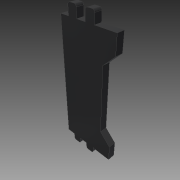
# Autodesk Inventor part: spool_stand_brace_middle_a
Saved by Autodesk Inventor 2014 (Build 180170000, 170)
## iProperties
Created: 2014-04-08
Part Number: spool_stand_brace_middle_a
Material: Plywood, Finish
Document SubType Name: Modeling
Designer: buben
Density: 0.552 g/cm^3
Appearance: Plywood - New
Author: buben
Autodesk Inventor part; units mm, degrees
ref_plane "YZ Plane" through (0, 0, 0) normal (1, 0, 0) x (0, 1, 0)
ref_plane "XZ Plane" through (0, 0, 0) normal (0, 1, 0) x (-1, 0, 0)
ref_plane "XY Plane" through (0, 0, 0) normal (0, 0, 1) x (1, 0, 0)
sketch "Sketch1" plane through (0, 0, 0) normal (0, 1, 0) x (-1, 0, 0)
  line L0 (0, 0) -> (-40, 0)
  line L1 (-40, 0) -> (-40, -110)
  line L2 (-40, -110) -> (0, -110)
  line L3 (0, -110) -> (0, 0)
  dimension "d0" = 110
  dimension "d1" = 40
  constraints: 8 end point, 2 parallel, 1 horizontal, 1 perpendicular
  measures "d0" distance of L2.end L0.start
  measures "d1" distance of L0.start L0.end
extrude "Extrusion1" add sketch "Sketch1" along normal blind 6.5
sketch "Sketch2" plane through (0, 6.5, 0) normal (0, 1, 0) x (1, 0, 0)
  line L0 (40, 0) -> (40, 110) projected
  line L1 (40, 110) -> (0, 110) projected
  line L2 (0, 110) -> (0, 0) projected
  line L3 (8, 110) -> (16, 110)
  line L4 (16, 110) -> (16, 114.5)
  line L5 (14, 116.5) -> (10, 116.5)
  line L6 (8, 114.5) -> (8, 110)
  line L7 (24, 110) -> (32, 110)
  line L8 (32, 110) -> (32, 114.5)
  line L9 (30, 116.5) -> (26, 116.5)
  line L10 (24, 114.5) -> (24, 110)
  arc A0 (10, 116.5) -> (8, 114.5) centre (10, 114.5) ccw
  arc A1 (16, 114.5) -> (14, 116.5) centre (14, 114.5) ccw
  arc A2 (26, 116.5) -> (24, 114.5) centre (26, 114.5) ccw
  arc A3 (32, 114.5) -> (30, 116.5) centre (30, 114.5) ccw
  line L11 (8, 112.25) -> (0, 112.25) construction
  line L12 (16, 112.25) -> (24, 112.25) construction
  line L13 (32, 112.25) -> (40, 112.25) construction
  line L14 (0, 55) -> (40, 55) construction
  line L15 (0, 0) -> (40, 0) projected
  line L16 (40, 0) -> (40, 110) projected
  line L17 (40, 110) -> (0, 110) projected
  line L18 (0, 110) -> (0, 0) projected
  line L19 (8, 0) -> (16, 0)
  line L20 (16, 0) -> (16, -7.5)
  line L21 (14, -9.5) -> (10, -9.5)
  line L22 (8, -7.5) -> (8, 0)
  line L23 (24, 0) -> (32, 0)
  line L24 (32, 0) -> (32, -7.5)
  line L25 (30, -9.5) -> (26, -9.5)
  line L26 (24, -7.5) -> (24, 0)
  arc A4 (8, -7.5) -> (10, -9.5) centre (10, -7.5) ccw
  arc A5 (14, -9.5) -> (16, -7.5) centre (14, -7.5) ccw
  arc A6 (24, -7.5) -> (26, -9.5) centre (26, -7.5) ccw
  arc A7 (30, -9.5) -> (32, -7.5) centre (30, -7.5) ccw
  dimension "d4" = 2
  dimension "d5" = 8
  dimension "d6" = 8
  dimension "d7" = 6.5
  dimension "d10" = 2
  dimension "d11" = 9.5
  constraints: 40 end point, 16 point on circle, 16 tangent, 9 collinear, 8 centre point, 8 parallel, 6 equal radius, 6 midpoint, 5 perpendicular, 4 horizontal, 4 point on line, 2 vertical alignment
  measures "d4" radius of A0
  measures "d5" distance between parallel lines of L4 L6
  measures "d6" distance between parallel lines of L8 L10
  measures "d7" distance between parallel lines of L3 L5
  measures "d10" radius of A4
  measures "d11" distance between parallel lines of L15 L21
extrude "Extrusion3" add sketch "Sketch2" against normal blind 6.5 contours L24 A7 L25 A6 L26 L15 | L1 L10 A2 L9 A3 L8 | L20 A5 L21 A4 L22 L15 | L1 L6 A0 L5 A1 L4
sketch "Sketch3" plane through (0, 0, 0) normal (0, -1, 0) x (1, 0, 0)
  line L0 (0, -110) -> (0, 0) projected
  line L1 (40, 0) -> (40, -110) projected
  line L2 (8, 7.5) -> (8, 0) projected
  line L3 (40, 0) -> (50, 0)
  line L4 (50, 0) -> (50, -15)
  line L5 (50, -15) -> (40, -25)
  line L6 (40, -85) -> (50, -95)
  line L7 (50, -95) -> (50, -110)
  line L8 (50, -110) -> (40, -110)
  line L9 (40, -85) -> (40, -110)
  line L10 (40, 0) -> (40, -25)
  dimension "d14" = 10
  dimension "d15" = 15
  dimension "d16" = 45
  dimension "d17" = 15
  constraints: 16 end point, 4 collinear, 4 perpendicular, 2 point on line, 1 parallel
  measures "d14" distance of L1.start L3.end
  measures "d15" distance of L3.end L4.end
  measures "d16" angle of L1 L5
  measures "d17" distance of L6.end L7.end
extrude "Extrusion4" add sketch "Sketch3" against normal blind 6.5
equation "\"d6\" = d5"
equation "\"d17\" = d15"
body "Solid1"
